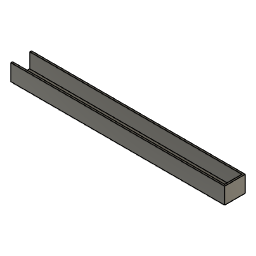
LOST-Wheel cord guard (Autodesk Fusion 360 design; units mm, degrees)
Autodesk Fusion 360 part; units mm, degrees
note: some values were not read from the file. Set by a fixed rule: which sketch regions a step uses.
sketch "Sketch1" plane through (0, 0, 0) normal (0, 0, 1) x (1, 0, 0)
  line L0 (76.5, 1.75) -> (84, 1.75)
  line L1 (84, 1.75) -> (84, 12.25)
  line L2 (84, 12.25) -> (76.5, 12.25)
  line L3 (76.5, 12.25) -> (76.5, 1.75)
  line L4 (85, -2.75) -> (72.5, -2.75)
  line L5 (72.5, -2.75) -> (72.5, 13.25)
  line L6 (72.5, 13.25) -> (85, 13.25)
  line L7 (85, 13.25) -> (85, -2.75)
  line L8 (85, -2.75) -> (72.5, 13.25) construction
  line L9 (72.5, -2.75) -> (85, 13.25) construction
  line L10 (85, 13.25) -> (-45, 13.25)
  line L11 (-45, 13.25) -> (-45, 0.75)
  line L12 (-45, 0.75) -> (85, 0.75)
  line L13 (85, 0.75) -> (85, 13.25)
  line L14 (76.5, 12.25) -> (-45, 12.25)
  line L15 (-45, 12.25) -> (-45, 13.25)
  line L16 (-45, 13.25) -> (76.5, 13.25)
  line L17 (76.5, 13.25) -> (76.5, 12.25)
  line L18 (76.5, 1.75) -> (-45, 1.75)
  line L19 (-45, 1.75) -> (-45, 0.75)
  line L20 (-45, 0.75) -> (76.5, 0.75)
  line L21 (76.5, 0.75) -> (76.5, 1.75)
  point P0 (78.75, 5.25)
  dimension "d1" = 7.5
  dimension "d2" = 10.5
  dimension "d3" = 12.5
  dimension "d4" = 16
  dimension "d5" = 130
  dimension "d6" = 12.5
  dimension "d11" = 1
  dimension "d12" = 1
  constraint horizontal L0
  constraint vertical L1
  constraint horizontal L2
  constraint vertical L3
  constraint horizontal L4
  constraint perpendicular L4 L5
  constraint parallel L4 L6
  constraint parallel L5 L7
  constraint coincident L8 P0
  constraint coincident L9 P0
  constraint horizontal L10
  constraint vertical L11
  constraint horizontal L12
  constraint vertical L13
  constraint horizontal L14
  constraint vertical L15
  constraint horizontal L16
  constraint vertical L17
  constraint horizontal L18
  constraint vertical L19
  constraint horizontal L20
  constraint vertical L21
  measures "d1" distance of L0.start L0.end
  measures "d2" distance of L0.start L2.end
  measures "d3" distance of L5.end L6.end
  measures "d4" distance of L4.end L5.end
  measures "d5" distance of L6.end L10.end
  measures "d6" distance of L6.end L12.end
  measures "d11" distance of L10 L14
  measures "d12" distance of L1 L13
extrude "Extrude1" add sketch "Sketch1" along normal blind 10 contours L5 L12 L18 L20 L21 | L0 L1 L2 L6 L7 L10 L12 L13 L17 L21 | L5 L6 L10 L14 L16 L17 | L5 L11 L12 L18 L19 L20 | L5 L10 L11 L14 L15 L16
extrude "Extrude2" add sketch "Sketch1" along normal blind 1 contours L3 L5 L14 L18 | L5 L11 L14 L18
